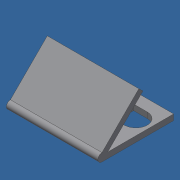
# Autodesk Inventor part: CameraBracket
Saved by Autodesk Inventor 2021 (Build 250183000, 183)
## iProperties
Created: 2022-09-10
Part Number: CameraBracket
Material: Generic
Document SubType Name: Modeling
Designer: Nathann
Density: 1 g/cm^3
Appearance: Default
Author: Nathann
Autodesk Inventor part; units mm, degrees
ref_plane "YZ Plane" through (0, 0, 0) normal (1, 0, 0) x (0, 1, 0)
ref_plane "XZ Plane" through (0, 0, 0) normal (0, 1, 0) x (-1, 0, 0)
ref_plane "XY Plane" through (0, 0, 0) normal (0, 0, 1) x (1, 0, 0)
sketch "Sketch1" plane through (0, 0, 0) normal (0, 1, 0) x (-1, 0, 0)
  circle A0 centre (0, 0) radius 10
  circle A1 centre (-54, 0) radius 10
  line L0 (-54, -10) -> (0, -10)
  line L1 (0, 10) -> (-54, 10)
  circle A2 centre (-16, -6.1173) radius 1.25
  circle A3 centre (-37, -6.1173) radius 1.25
  circle A4 centre (-37, 6.3827) radius 1.25
  circle A5 centre (-16, 6.3827) radius 1.25
  line L2 (-11, -10) -> (-11, 10)
  line L3 (-21, 10) -> (-21, -10)
  line L4 (-32, -10) -> (-32, 10)
  line L5 (-42, -10) -> (-42, 10)
  line L6 (13, -20) -> (-67, -20)
  line L7 (-67, -20) -> (-67, 20)
  line L8 (-67, 20) -> (13, 20)
  line L9 (13, 20) -> (13, -20)
  dimension "d0" = 20
  dimension "d1" = 20
  dimension "d2" = 54
  dimension "d3" = 21
  dimension "d4" = 12.5
  dimension "d5" = 12.5
  dimension "d6" = 21
  dimension "d7" = 2.5
  dimension "d8" = 2.5
  dimension "d9" = 2.5
  dimension "d10" = 2.5
  dimension "d11" = 5
  dimension "d12" = 5
  dimension "d13" = 5
  dimension "d14" = 5
  dimension "d15" = 11
  dimension "d16" = 11
  dimension "d17" = 40
  dimension "d18" = 80
  dimension "d19" = 13
  dimension "d20" = 20
  constraints: 20 end point, 8 point on line, 6 centre point, 5 perpendicular, 4 point on circle, 3 horizontal, 3 tangent, 2 parallel, 1 coincident, 1 horizontal alignment, 1 vertical alignment
  measures "d0" diameter of A1
  measures "d1" diameter of A0
  measures "d2" distance of A1.centre point (0, 0)
  measures "d3" distance of A3.centre A2.centre
  measures "d4" distance of A5.centre A2.centre
  measures "d5" distance of A3.centre A4.centre
  measures "d6" distance of A5.centre A4.centre
  measures "d7" diameter of A2
  measures "d8" diameter of A3
  measures "d9" diameter of A4
  measures "d10" diameter of A5
  measures "d11" distance from line of L2 A5.centre
  measures "d12" distance from line of L3 A5.centre
  measures "d13" distance from line of L4 A4.centre
  measures "d14" distance from line of L5 A4.centre
  measures "d15" distance between parallel lines of L4 L3
  measures "d16" distance from line of point (0, 0) L2
  measures "d17" distance of L6.end L7.end
  measures "d18" distance of L6.start L6.end
  measures "d19" distance from line of L7 A1.centre
  measures "d20" distance from line of L8 A1.centre
extrude "Extrusion1" add sketch "Sketch1" along normal blind 5 contours L2 L0 L3 L1 | L4 L0 L5 L1 | L6 L7 L8 L9
sketch "Sketch2" plane through (67, 0, 20) normal (1, 0, 0) x (0, 0, -1)
  line L0 (0, 0) -> (-17.6204, 0)
  line L1 (-17.6204, 0) -> (-17.6204, 5)
  line L2 (-17.6204, 5) -> (0, 5)
  line L3 (0, 5) -> (0, 0)
  line L4 (-17.6204, 5) -> (13.1355, 35.7559)
  line L5 (13.1355, 35.7559) -> (9.5999, 39.2914)
  line L6 (9.5999, 39.2914) -> (-22.6204, 7.0711)
  line L7 (-22.6204, 7.0711) -> (-22.6204, 0)
  line L8 (-22.6204, 0) -> (-17.6204, 0)
  circle A0 centre (-22.6204, 3.5355) radius 3.5355
  point P0 (-22.6204, 0)
  dimension "d23" = 45
  dimension "d24" = 5
  dimension "d25" = 5
  constraints: 18 end point, 4 perpendicular, 2 parallel, 1 coincident, 1 horizontal, 1 midpoint, 1 point on line, 1 vertical, 3 other
  measures "d23" angle of L2 L4
  measures "d24" distance between parallel lines of L0 L2
  measures "d25" distance between parallel lines of L6 L4
extrude "Extrusion2" add sketch "Sketch2" against normal blind 80
sketch "Sketch3" plane through (0, 5, 0) normal (0, 1, 0) x (1, 0, 0)
  line L0 (12, -20) -> (42, -20)
  line L1 (42, -20) -> (42, -30)
  line L2 (42, -30) -> (12, -30)
  line L3 (12, -30) -> (12, -20)
  line L4 (-13, 20) -> (-13, -37.6204) projected
  line L5 (11, -10) -> (0, -10) projected
  point P0 (0, 0)
  dimension "d28" = 30
  dimension "d29" = 10
  dimension "d30" = 25
  dimension "d31" = 10
  constraints: 8 end point, 2 parallel, 1 horizontal, 1 perpendicular
  measures "d28" distance of L0.start L0.end
  measures "d29" distance of L2.end L0.start
  measures "d30" distance between parallel lines of L3 L4
  measures "d31" distance between parallel lines of L0 L5
extrude "Extrusion3" cut sketch "Sketch3" against normal blind 80
sketch "Sketch4" plane through (67, 5, 37.6204) normal (0, -0.7071068, -0.7071068) x (-1, 0, 0)
  circle A0 centre (73.7126, 34.5024) radius 2.2513
  circle A1 centre (10, 33.4954) radius 2.25
  line L0 (0, 0) -> (0, 43.4954) projected
  line L1 (0, 43.4954) -> (80, 43.4954) projected
  circle A2 centre (70, 33.4954) radius 2.25
  line L2 (80, 37.2082) -> (80, -7.0711) projected
  point P0 (67, 23.0661)
  point P1 (71.5496, 35.1267)
  point P2 (72.1615, 32.8706)
  dimension "d34" = 10
  dimension "d35" = 10
  dimension "d36" = 4.5
  dimension "d37" = 10
  dimension "d38" = 10
  dimension "d39" = 4.5
  constraints: 3 centre point
  measures "d34" distance from line of L0 A1.centre
  measures "d35" distance from line of L1 A1.centre
  measures "d36" diameter of A1
  measures "d37" distance from line of L1 A2.centre
  measures "d38" distance from line of L2 A2.centre
  measures "d39" diameter of A2
extrude "Extrusion4" cut sketch "Sketch4" against normal blind 80 contours A0 A2 | A1 picked at (74.6057, 34.8394)
equation "\"d5\" = d4"
equation "\"d6\" = d3"
equation "\"d39\" = d36"
body "Solid1"
